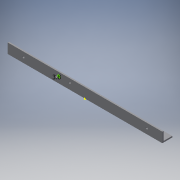
# Autodesk Inventor part: L
Saved by Autodesk Inventor 2018 (Build 220112000, 112)
## iProperties
Created: 2018-06-01
Part Number: L
Material: Generic
Document SubType Name: Modeling
Designer: David
Density: 1 g/cm^3
Appearance: Default
Author: David
Autodesk Inventor part; units mm, degrees
ref_plane "YZ Plane" through (0, 0, 0) normal (1, 0, 0) x (0, 1, 0)
ref_plane "XZ Plane" through (0, 0, 0) normal (0, 1, 0) x (-1, 0, 0)
ref_plane "XY Plane" through (0, 0, 0) normal (0, 0, 1) x (1, 0, 0)
sketch "Sketch1" plane through (0, 0, 0) normal (0, 0, 1) x (1, 0, 0)
  line L0 (117.25, -7.54) -> (-117.25, -7.54)
  line L1 (-117.25, -7.54) -> (-117.25, 7.54)
  line L2 (-117.25, 7.54) -> (117.25, 7.54)
  line L3 (117.25, 7.54) -> (117.25, -7.54)
  line L4 (117.25, -7.54) -> (-117.25, 7.54) construction
  line L5 (-117.25, -7.54) -> (117.25, 7.54) construction
  point P0 (0, 0)
  dimension "d0" = 234.5
  dimension "d1" = 15.08
  constraints: 12 end point, 2 midpoint, 2 parallel, 1 horizontal, 1 perpendicular
  measures "d0" distance of L1.end L2.end
  measures "d1" distance of L0.end L1.end
extrude "Extrusion1" add sketch "Sketch1" along normal blind 2.05
sketch "Sketch2" plane through (0, 0, 2.05) normal (0, 0, 1) x (1, 0, 0)
  line L0 (-117.25, -7.54) -> (117.25, -7.54) projected
  line L1 (117.25, -7.54) -> (117.25, 7.54) projected
  line L2 (-117.25, -7.54) -> (117.25, -7.54)
  line L3 (117.25, -7.54) -> (117.25, -5.49)
  line L4 (117.25, -5.49) -> (-117.25, -5.49)
  line L5 (-117.25, -5.49) -> (-117.25, -7.54)
  point P0 (0, 0)
  dimension "d4" = 2.05
  constraints: 8 end point, 2 parallel, 1 horizontal, 1 perpendicular, 1 point on line
  measures "d4" distance of L3.end L2.end
extrude "Extrusion2" add sketch "Sketch2" along normal blind 13.03
sketch "Sketch3" plane through (-117.25, -5.49, 2.05) normal (0, 1, 0) x (1, 0, 0)
  circle A0 centre (23.75, -5.95) radius 1.6
  circle A1 centre (210.75, -5.95) radius 1.6
  line L0 (117.25, 2.05) -> (117.25, -13.2508)
  line L1 (0, 2.05) -> (234.5, 2.05) projected
  dimension "d7" = 93.5
  dimension "d8" = 93.5
  dimension "d9" = 8
  dimension "d10" = 8
  dimension "d13" = 3.2
  dimension "d14" = 3.2
  constraints: 2 centre point, 2 end point, 1 vertical
  measures "d7" distance from line of A0.centre L0
  measures "d8" distance from line of L0 A1.centre
  measures "d9" distance from line of L1 A1.centre
  measures "d10" distance from line of L1 A0.centre
  measures "d13" diameter of A0
  measures "d14" diameter of A1
extrude "Extrusion3" cut sketch "Sketch3" against normal blind 2.05
sketch "Sketch4" plane through (-117.25, -7.54, 0) normal (0, -1, 0) x (1, 0, 0)
  circle A0 centre (77.4621, 9.6496) radius 1.9
  point P0 (117.25, 0)
  dimension "d15" = 3.8
  constraints: 1 centre point
  measures "d15" diameter of A0
sketch "Sketch5" plane through (0, 0, 2.05) normal (0, 0, 1) x (1, 0, 0)
  circle A0 centre (93.5, 2.51) radius 2.1
  circle A1 centre (-93.4, 2.51) radius 2.1
  line L0 (117.25, -5.49) -> (-117.25, -5.49) projected
  point P0 (0, 0)
  dimension "d18" = 4.2
  dimension "d19" = 4.2
  dimension "d20" = 8
  dimension "d21" = 8
  dimension "d22" = 93.5
  dimension "d23" = 93.4
  constraints: 2 centre point
  measures "d18" diameter of A0
  measures "d19" diameter of A1
  measures "d20" distance from line of L0 A0.centre
  measures "d21" distance from line of L0 A1.centre
  measures "d22" horizontal distance of A0.centre point (0, 0)
  measures "d23" horizontal distance of point (0, 0) A1.centre
extrude "Extrusion5" cut sketch "Sketch5" against normal blind 2.05
sketch "Sketch6" plane through (-117.25, -5.49, 2.05) normal (0, 1, 0) x (1, 0, 0)
  circle A0 centre (73.0521, -4.95) radius 1.75 projected
  point P0 (117.25, 2.05)
extrude "Extrusion6" cut sketch "Sketch6" against normal blind 3
sketch "Sketch7" plane through (-117.25, -5.49, 2.05) normal (0, 1, 0) x (1, 0, 0)
  circle A0 centre (73.0521, -4.95) radius 1.75 projected
  circle A1 centre (23.75, -5.95) radius 1.6 projected
  circle A2 centre (210.75, -5.95) radius 1.6 projected
  line L0 (0, 0) -> (234.5, 0) projected
  line L1 (0, 0) -> (0, -13.03) projected
  line L2 (234.5, -13.03) -> (0, -13.03) projected
  line L3 (234.5, 0) -> (234.5, -13.03) projected
  circle A3 centre (93.9521, -7.45) radius 1.6 projected
  point P0 (117.25, 2.05)
extrude "Extrusion7" cut sketch "Sketch7" against normal blind 10 contours A3
body "Solid1"
